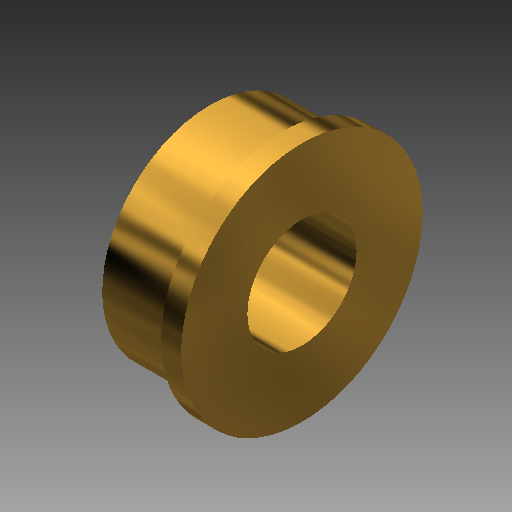
# Autodesk Inventor part: Clutch Bearing
Saved by Autodesk Inventor 2017 (Build 210135000, 135)
## iProperties
Created: 2012-08-06
Part Number: Clutch Bearing
Material: Brass, Soft Yellow
Document SubType Name: Modeling
Designer: John
Mass: 1.20107 g
Surface Area: 2.76966 cm^2
Volume: 0.141803 cm^3
Density: 8.47 g/cm^3
Appearance: Brass - Satin
Author: John
Autodesk Inventor part; units mm, degrees
ref_plane "YZ Plane" through (0, 0, 0) normal (1, 0, 0) x (0, 1, 0)
ref_plane "XZ Plane" through (0, 0, 0) normal (0, 1, 0) x (-1, 0, 0)
ref_plane "XY Plane" through (0, 0, 0) normal (0, 0, 1) x (1, 0, 0)
sketch "Sketch1" plane through (0, 0, 0) normal (1, 0, 0) x (0, 1, 0)
  circle A0 centre (0, 0) radius 4.7625
  dimension "d0" = 9.525
  constraints: 1 centre point, 1 coincident
  measures "d0" diameter of A0
extrude "Extrusion1" add sketch "Sketch1" along normal blind 3.175
sketch "Sketch2" plane through (3.175, 0, 0) normal (1, 0, 0) x (0, 0, -1)
  circle A0 centre (0, 0) radius 4.7625 projected
  circle A1 centre (0, 0) radius 5.334
  dimension "d4" = 10.668
  constraints: 1 centre point, 1 coincident
  measures "d4" diameter of A1
extrude "Extrusion2" add sketch "Sketch2" along normal blind 0.889 contours A0 | A1
sketch "Sketch3" plane through (4.064, 0, 0) normal (1, 0, 0) x (0, 0, -1)
  circle A0 centre (0, 0) radius 5.334 projected
hole "Hole1" at (4.064, 0, 0) direction (-1, 0, 0) diameter 4.826 end through all
body "Solid1"
